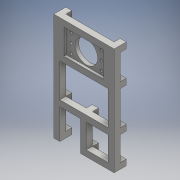
# Autodesk Inventor part: sideFrame
Saved by Autodesk Inventor 2016 (Build 200138000, 138)
## iProperties
Created: 2016-06-04
Part Number: sideFrame
Material: Generic
Document SubType Name: Modeling
Designer: hesaon
Density: 1 g/cm^3
Appearance: Default
Author: hesaon
Autodesk Inventor part; units mm, degrees
ref_plane "YZ Plane" through (0, 0, 0) normal (1, 0, 0) x (0, 1, 0)
ref_plane "XZ Plane" through (0, 0, 0) normal (0, 1, 0) x (-1, 0, 0)
ref_plane "XY Plane" through (0, 0, 0) normal (0, 0, 1) x (1, 0, 0)
sketch "Sketch1" plane through (0, 0, 0) normal (0, 1, 0) x (-1, 0, 0)
  line L0 (0, 0) -> (100, 0)
  line L1 (100, 0) -> (100, -178)
  line L2 (0, -178) -> (0, 0)
  line L3 (90, -10) -> (10, -10)
  line L4 (90, -52) -> (10, -52)
  line L5 (90, -62) -> (10, -62)
  line L6 (90, -52) -> (90, -10)
  line L7 (10, -10) -> (10, -52)
  line L8 (90, -118) -> (10, -118)
  line L9 (90, -168) -> (90, -128)
  line L10 (90, -118) -> (90, -62)
  line L11 (10, -62) -> (10, -118)
  line L12 (10, -128) -> (10, -168)
  line L13 (100, -178) -> (90, -178)
  line L14 (10, -178) -> (0, -178)
  line L15 (90, -168) -> (90, -178)
  line L16 (10, -168) -> (46, -168)
  line L17 (56, -168) -> (56, -178)
  line L18 (56, -178) -> (10, -178)
  line L19 (56, -168) -> (56, -128)
  line L20 (46, -128) -> (46, -168)
  line L21 (90, -128) -> (56, -128)
  line L22 (46, -128) -> (10, -128)
  dimension "thickness" = 10
  dimension "d3" = 10
  dimension "d4" = 10
  dimension "d8" = 10
  dimension "motor" = 42
  dimension "d10" = 10
  dimension "d11" = 10
  dimension "d27" = 10
  dimension "batterywidth" = 56
  dimension "d31" = 80
  dimension "suspensionWidth" = 40
  dimension "d33" = 10
  dimension "d34" = 10
  dimension "suspensionHeight" = 34
  dimension "d36" = 10
  dimension "d38" = 10
  dimension "d39" = 40
  dimension "d40" = 40
  dimension "d41" = 36
  constraints: 46 end point, 21 perpendicular, 12 parallel, 3 horizontal, 2 point on line, 1 vertical
  measures "thickness" distance from line of L1 L3.start
  measures "d3" distance from line of L0 L3.start
  measures "d4" distance from line of L2 L3.end
  measures "d8" distance of L5.start L4.start
  measures "motor" distance of L4.start L3.start
  measures "d10" distance from line of L2 L5.end
  measures "d11" distance of L5.end L4.end
  measures "d27" distance of L9.end L8.start
  measures "batterywidth" distance of L5.start L8.start
  measures "d31" distance of L12.start L9.end
  measures "suspensionWidth" distance of L9.start L9.end
  measures "d33" distance of L13.end L9.start
  measures "d34" distance of L17.end L17.start
  measures "suspensionHeight" distance of L17.end L13.end
  measures "d36" distance of L16.end L17.start
  measures "d38" distance from line of L2 L12.end
  measures "d39" distance of L12.end L12.start
  measures "d40" distance of L17.start L19.end
  measures "d41" distance of L12.end L16.end
extrude "Extrusion2" add sketch "Sketch1" along normal blind 10
sketch "Sketch2" plane through (0, 10, 0) normal (0, 1, 0) x (1, 0, 0)
  line L0 (-100, 0) -> (-90, 0)
  line L1 (-90, 0) -> (-90, 10)
  line L2 (-90, 10) -> (-100, 10)
  line L3 (-100, 10) -> (-100, 0)
  line L4 (-10, 52) -> (-10, 10) projected
  line L5 (0, 0) -> (-10, 0)
  line L6 (-10, 0) -> (-10, 10)
  line L7 (-10, 10) -> (0, 10)
  line L8 (0, 10) -> (0, 0)
  line L9 (-100, 178) -> (-100, 0) projected
  line L10 (-100, 0) -> (0, 0) projected
  line L11 (-100, 52) -> (-90, 52)
  line L12 (-90, 52) -> (-90, 62)
  line L13 (-90, 62) -> (-100, 62)
  line L14 (-100, 62) -> (-100, 52)
  line L15 (-90, 52) -> (-10, 52) projected
  line L16 (-10, 52) -> (0, 52)
  line L17 (0, 52) -> (0, 62)
  line L18 (0, 62) -> (-10, 62)
  line L19 (-10, 62) -> (-10, 52)
  line L20 (-90, 10) -> (-90, 52) projected
  line L21 (-100, 118) -> (-90, 118)
  line L22 (-90, 118) -> (-90, 128)
  line L23 (-90, 128) -> (-100, 128)
  line L24 (-100, 128) -> (-100, 118)
  line L25 (-100, 168) -> (-90, 168)
  line L26 (-90, 168) -> (-90, 178)
  line L27 (-90, 178) -> (-100, 178)
  line L28 (-100, 178) -> (-100, 168)
  line L29 (-56, 128) -> (-90, 128) projected
  line L30 (-90, 178) -> (-100, 178) projected
  line L31 (-56, 118) -> (-46, 118)
  line L32 (-46, 118) -> (-46, 128)
  line L33 (-46, 128) -> (-56, 128)
  line L34 (-56, 128) -> (-56, 118)
  line L35 (-56, 178) -> (-56, 128) projected
  line L36 (-90, 118) -> (-10, 118) projected
  line L37 (-56, 178) -> (-46, 178)
  line L38 (-46, 178) -> (-46, 168)
  line L39 (-46, 168) -> (-56, 168)
  line L40 (-56, 168) -> (-56, 178)
  line L41 (0, 178) -> (-56, 178) projected
  line L42 (-10, 168) -> (0, 168)
  line L43 (0, 168) -> (0, 178)
  line L44 (0, 178) -> (-10, 178)
  line L45 (-10, 178) -> (-10, 168)
  line L46 (0, 0) -> (0, 178) projected
  line L47 (-10, 118) -> (0, 118)
  line L48 (0, 118) -> (0, 128)
  line L49 (0, 128) -> (-10, 128)
  line L50 (-10, 128) -> (-10, 118)
  line L51 (-10, 128) -> (-46, 128) projected
  dimension "d44" = 10
  dimension "d45" = 10
  dimension "d47" = 10
  dimension "d50" = 10
  dimension "d51" = 10
  dimension "d52" = 10
  dimension "d53" = 10
  dimension "d54" = 10
  dimension "d55" = 10
  dimension "d56" = 10
  dimension "d57" = 10
  dimension "d58" = 10
  dimension "d59" = 10
  dimension "d60" = 10
  dimension "d61" = 10
  dimension "d62" = 10
  dimension "d63" = 10
  dimension "d64" = 10
  dimension "d65" = 10
  constraints: 80 end point, 22 collinear, 21 parallel, 10 horizontal, 10 perpendicular
  measures "d44" distance of L2.end L1.end
  measures "d45" distance of L1.end L0.end
  measures "d47" distance of L5.end L4.end
  measures "d50" distance of L13.end L12.end
  measures "d51" distance of L12.end L11.end
  measures "d52" distance of L18.end L17.end
  measures "d53" distance of L17.end L16.end
  measures "d54" distance of L23.end L22.end
  measures "d55" distance of L22.end L21.end
  measures "d56" distance of L27.end L26.end
  measures "d57" distance of L26.end L25.end
  measures "d58" distance of L33.end L32.end
  measures "d59" distance of L32.end L31.end
  measures "d60" distance of L38.end L39.end
  measures "d61" distance of L37.end L38.end
  measures "d62" distance of L44.end L43.end
  measures "d63" distance of L43.end L42.end
  measures "d64" distance of L49.end L48.end
  measures "d65" distance of L48.end L47.end
extrude "Extrusion3" add sketch "Sketch2" along normal blind 10 contours L3 L2 L1 L0 | L6 L7 L8 L5 | L9 L13 L12 L11 | L19 L18 L17 L16 | L9 L23 L22 L21 | L34 L33 L32 L31 | L47 L50 L49 L46 | L35 L37 L38 L39 | L42 L45 L41 L43 | L27 L26 L25 L9
sketch "Sketch6" plane through (0, 0, 0) normal (0, -1, 0) x (1, 0, 0)
  line L0 (-90, -10) -> (-83, -10)
  line L1 (-83, -10) -> (-83, -52)
  line L2 (-83, -52) -> (-90, -52)
  line L3 (-90, -52) -> (-90, -10)
  line L4 (-90, -52) -> (-90, -10) projected
  line L5 (-90, -10) -> (-10, -10) projected
  line L6 (-10, -52) -> (-90, -52) projected
  line L7 (-17, -10) -> (-10, -10)
  line L8 (-10, -10) -> (-10, -52)
  line L9 (-10, -52) -> (-17, -52)
  line L10 (-17, -52) -> (-17, -10)
  line L11 (-10, -10) -> (-10, -52) projected
  point P0 (0, 0)
  dimension "motorFixtureHeight" = 66
  dimension "d72" = 7
  constraints: 16 end point, 6 collinear, 4 parallel, 2 horizontal, 2 perpendicular
  measures "motorFixtureHeight" distance of L7.start L0.end
  measures "d72" distance of L5.end L7.start
extrude "Extrusion5" add sketch "Sketch6" against normal blind 10 contours L0 L1 L2 L3 | L5 L8 L6 L10
sketch "Sketch7" plane through (0, 10, 0) normal (0, 1, 0) x (1, 0, 0)
  line L0 (-83, 10) -> (-17, 10)
  line L1 (-17, 10) -> (-17, 52)
  line L2 (-17, 52) -> (-83, 52)
  line L3 (-83, 52) -> (-83, 10)
  line L4 (-83, 10) -> (-83, 52) projected
  line L5 (-83, 52) -> (-17, 52) projected
  line L6 (-17, 52) -> (-17, 10) projected
  line L7 (-17, 10) -> (-83, 10) projected
  circle A0 centre (-50, 31) radius 18.75
  circle A1 centre (-75, 16) radius 2.1
  circle A2 centre (-25, 31) radius 2.1
  circle A3 centre (-75, 46) radius 2.1
  circle A4 centre (-25, 16) radius 2.1
  circle A5 centre (-25, 46) radius 2.1
  circle A6 centre (-75, 31) radius 2.1
  point P0 (0, 0)
  dimension "d75" = 37.5
  dimension "d77" = 21
  dimension "d78" = 33
  dimension "d79" = 4.2
  dimension "d80" = 4.2
  dimension "d82" = 4.2
  dimension "d83" = 4.2
  dimension "d84" = 4.2
  dimension "d85" = 4.2
  dimension "d86" = 25
  dimension "d87" = 0
  dimension "d88" = 25
  dimension "d89" = 15
  dimension "d90" = 25
  dimension "d91" = 15
  dimension "d92" = 15
  dimension "d93" = 25
  dimension "d94" = 25
  dimension "d95" = 0
  dimension "d96" = 25
  dimension "d97" = 15
  constraints: 8 end point, 7 centre point, 4 collinear, 2 parallel, 1 horizontal, 1 perpendicular
  measures "d75" diameter of A0
  measures "d77" distance from line of L0 A0.centre
  measures "d78" distance from line of L1 A0.centre
  measures "d79" diameter of A1
  measures "d80" diameter of A2
  measures "d82" diameter of A3
  measures "d83" diameter of A4
  measures "d84" diameter of A5
  measures "d85" diameter of A6
  measures "d86" distance of A6.centre A0.centre
  measures "d87" vertical distance of A0.centre A6.centre
  measures "d88" horizontal distance of A0.centre A1.centre
  measures "d89" distance of A6.centre A1.centre
  measures "d90" horizontal distance of A0.centre A3.centre
  measures "d91" distance of A6.centre A3.centre
  measures "d92" vertical distance of A0.centre A4.centre
  measures "d93" horizontal distance of A0.centre A4.centre
  measures "d94" distance of A0.centre A2.centre
  measures "d95" vertical distance of A0.centre A2.centre
  measures "d96" horizontal distance of A0.centre A5.centre
  measures "d97" distance of A5.centre A2.centre
extrude "Extrusion6" add sketch "Sketch7" against normal blind 6
equation "\"d3\" = thickness"
equation "\"d4\" = thickness"
equation "\"d8\" = thickness"
equation "\"d10\" = thickness"
equation "\"d11\" = thickness"
equation "\"d27\" = thickness"
equation "\"d33\" = thickness"
equation "\"d34\" = thickness"
equation "\"d36\" = thickness"
equation "\"d38\" = thickness"
equation "\"d39\" = suspensionWidth"
equation "\"d40\" = suspensionWidth"
equation "\"d42\" = thickness"
equation "\"d44\" = thickness"
equation "\"d50\" = thickness"
equation "\"d51\" = thickness"
equation "\"d52\" = thickness"
equation "\"d53\" = thickness"
equation "\"d54\" = thickness"
equation "\"d55\" = thickness"
equation "\"d56\" = thickness"
equation "\"d57\" = thickness"
equation "\"d58\" = thickness"
equation "\"d59\" = thickness"
equation "\"d60\" = thickness"
equation "\"d61\" = thickness"
equation "\"d62\" = thickness"
equation "\"d63\" = thickness"
equation "\"d64\" = thickness"
equation "\"d65\" = thickness"
equation "\"d66\" = thickness"
equation "\"d73\" = thickness"
equation "\"d77\" = 0.5 * motor"
body "Solid2"
